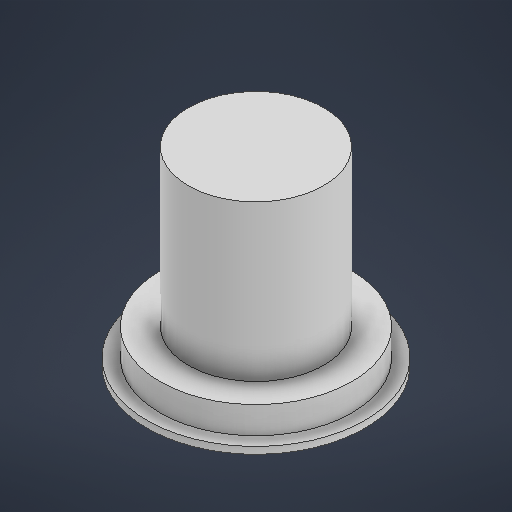
# Autodesk Inventor part: D28 - Forma
Saved by Autodesk Inventor 2026 (Build 300175000, 175)
## iProperties
Created: 2026-02-14
Part Number: D28 - Forma
Material: Všeobecné
Document SubType Name: Modeling
Designer: vadim
Density: 1 g/cm^3
Appearance: Výchozí
Author: vadim
Autodesk Inventor part; units mm, degrees
ref_plane "YZ Plane" through (0, 0, 0) normal (1, 0, 0) x (0, 1, 0)
ref_plane "XZ Plane" through (0, 0, 0) normal (0, 1, 0) x (-1, 0, 0)
ref_plane "XY Plane" through (0, 0, 0) normal (0, 0, 1) x (1, 0, 0)
sketch "Náčrt1" plane through (0, 0, 0) normal (0, 1, 0) x (-1, 0, 0)
  circle A0 centre (0, 0) radius 16.1
  circle A1 centre (0, 0) radius 14.175
  circle A2 centre (0, 0) radius 10
  circle A3 centre (0, 0) radius 8.5
  dimension "d0" = 32.2
  dimension "d1" = 28.35
  dimension "d2" = 20
  dimension "d3" = 1.5
  constraints: 4 centre point, 4 coincident
  measures "d0" diameter of A0
  measures "d1" diameter of A1
  measures "d2" diameter of A2
  measures "d3" radial gap between concentric circles of A2 A3
extrude "Vysunutí1" add sketch "Náčrt1" along normal blind 1 contours A0
extrude "Vysunutí2" add sketch "Náčrt1" along normal blind 5 contours A1
extrude "Vysunutí3" add sketch "Náčrt1" along normal blind 28 contours A2 | A3
extrude "Vysunutí4" cut sketch "Náčrt1" along normal blind 26.5 contours A3
fillet "Zaoblení1" radius 2.5 1 edges at (8.5, 26.5, 0)
chamfer "Zkosení1" distance 2 angle 45 1 edges at (8.5, 0, 0)
